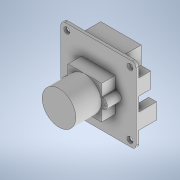
# Autodesk Inventor part: Trackingcam (Applied robotics)
Saved by Autodesk Inventor 2020 (Build 240168000, 168)
## iProperties
Created: 2021-02-21
Part Number: Trackingcam (Applied robotics)
Material: Типовые
Document SubType Name: Обычные детали
Designer: Антон
Density: 1 g/cm^3
Appearance: По умолчанию
Sheet Metal Rule: По умолчанию
Author: Антон
Autodesk Inventor part; units mm, degrees
ref_plane "YZ Plane" through (0, 0, 0) normal (1, 0, 0) x (0, 1, 0)
ref_plane "XZ Plane" through (0, 0, 0) normal (0, 1, 0) x (-1, 0, 0)
ref_plane "XY Plane" through (0, 0, 0) normal (0, 0, 1) x (1, 0, 0)
sketch "Эскиз1" plane through (0, 0, 0) normal (0, 0, 1) x (1, 0, 0)
  line L0 (0, 0) -> (38, 0)
  line L1 (38, 0) -> (38, 38)
  line L2 (38, 38) -> (0, 38)
  line L3 (0, 38) -> (0, 0)
  line L4 (0, 38) -> (3, 38)
  line L5 (3, 38) -> (3, 35)
  circle A0 centre (3, 35) radius 1.5
  circle A1 centre (35, 35) radius 1.5
  circle A2 centre (3, 3) radius 1.5
  circle A3 centre (35, 3) radius 1.5
  dimension "d0" = 38
  dimension "d1" = 38
  dimension "d2" = 3
  dimension "d3" = 3
  dimension "d4" = 3
  dimension "d7" = 32
  dimension "d10" = 32
  constraints: 12 end point, 4 centre point, 2 horizontal, 2 parallel, 2 perpendicular, 1 coincident, 1 point on line, 1 vertical, 6 other
  measures "d0" distance of L2.end L1.end
  measures "d1" distance of L1.end L0.end
  measures "d2" distance of L2.end L4.end
  measures "d3" distance of L4.end L5.end
  measures "d4" diameter of A0
  measures "d7" distance of A0.centre A1.centre
  measures "d10" distance of A0.centre A2.centre
extrude "Выдавливание1" add sketch "Эскиз1" along normal blind 1.4
fillet "Сопряжение1" radius 2 4 edges at (38, 38, 0.7) (38, 0, 0.7) (0, 0, 0.7) (0, 38, 0.7)
sketch "Эскиз2" plane through (0, 0, 1.4) normal (0, 0, 1) x (1, 0, 0)
  line L0 (2, 38) -> (10.5, 38)
  line L1 (36, 38) -> (2, 38) projected
  line L2 (10.5, 38) -> (10.5, 27.5)
  line L3 (10.5, 27.5) -> (27.5, 27.5)
  line L4 (27.5, 27.5) -> (27.5, 10.5)
  line L5 (27.5, 10.5) -> (10.5, 10.5)
  line L6 (10.5, 10.5) -> (10.5, 27.5)
  line L7 (27.5, 27.5) -> (27.5, 21.5)
  line L8 (27.5, 21.5) -> (30.5, 21.5)
  line L9 (30.5, 21.5) -> (30.5, 16.5)
  line L10 (30.5, 16.5) -> (27.5, 16.5)
  line L11 (27.5, 16.5) -> (27.5, 21.5)
  line L12 (10.5, 27.5) -> (10.5, 21.5)
  line L13 (10.5, 21.5) -> (7.5, 21.5)
  line L14 (7.5, 21.5) -> (7.5, 16.5)
  line L15 (7.5, 16.5) -> (10.5, 16.5)
  line L16 (10.5, 16.5) -> (10.5, 21.5)
  line L17 (30.5, 19) -> (29.5, 19)
  line L18 (7.5, 19) -> (8.5, 19)
  circle A0 centre (8.5, 19) radius 0.5
  circle A1 centre (29.5, 19) radius 0.5
  point P0 (0, 0)
  dimension "d20" = 8.5
  dimension "d21" = 10.5
  dimension "d22" = 17
  dimension "d23" = 17
  dimension "d83" = 6
  dimension "d84" = 3
  dimension "d85" = 5
  dimension "d86" = 6
  dimension "d87" = 3
  dimension "d88" = 5
  dimension "d89" = 1
  dimension "d90" = 1
  dimension "d91" = 1
  dimension "d92" = 1
  constraints: 36 end point, 6 parallel, 5 horizontal, 4 perpendicular, 3 point on line, 2 centre point, 2 coincident, 2 midpoint
  measures "d20" distance of L0.start L0.end
  measures "d21" distance of L0.end L2.end
  measures "d22" distance of L4.end L5.end
  measures "d23" distance of L3.end L4.end
  measures "d83" distance of L3.end L7.end
  measures "d84" distance of L9.end L10.end
  measures "d85" distance of L8.end L9.end
  measures "d86" distance of L2.end L12.end
  measures "d87" distance of L15.end L14.end
  measures "d88" distance of L14.end L13.end
  measures "d89" distance of L17.start L17.end
  measures "d90" distance of L18.start L18.end
  measures "d91" diameter of A0
  measures "d92" diameter of A1
extrude "Выдавливание2" add sketch "Эскиз2" along normal blind 7
sketch "Эскиз3" plane through (0, 0, 8.4) normal (0, 0, 1) x (1, 0, 0)
  line L0 (10.5, 27.5) -> (10.5, 10.5) projected
  line L1 (10.5, 19) -> (27.5, 19)
  line L2 (27.5, 27.5) -> (27.5, 10.5) projected
  circle A0 centre (19, 19) radius 8.5
  point P0 (0, 0)
  constraints: 3 midpoint, 2 end point, 1 horizontal alignment, 2 other
extrude "Выдавливание3" add sketch "Эскиз3" along normal blind 13
sketch "Эскиз4" plane through (0, 0, 0) normal (0, 0, -1) x (-1, 0, 0)
  arc A0 (-36, 38) -> (-38, 36) centre (-36, 36) ccw projected
  line L0 (-36, 38) -> (-29.25, 38)
  line L1 (-29.25, 38) -> (-29.25, 36)
  line L2 (-29.25, 36) -> (-8.75, 36)
  line L3 (-8.75, 36) -> (-8.75, 27)
  line L4 (-8.75, 27) -> (-29.25, 27)
  line L5 (-29.25, 27) -> (-29.25, 36)
  point P0 (0, 0)
  dimension "d41" = 6.75
  dimension "d42" = 2
  dimension "d43" = 20.5
  dimension "d44" = 9
  constraints: 12 end point, 2 horizontal, 2 parallel, 1 perpendicular, 1 tangent, 1 vertical
  measures "d41" distance of L0.start L0.end
  measures "d42" distance of L0.end L1.end
  measures "d43" distance of L3.end L4.end
  measures "d44" distance of L2.end L3.end
extrude "Выдавливание4" add sketch "Эскиз4" along normal blind 10
sketch "Эскиз5" plane through (0, 0, 0) normal (0, 0, -1) x (-1, 0, 0)
  arc A0 (-36, 38) -> (-38, 36) centre (-36, 36) ccw projected
  line L0 (-38, 36) -> (-38, 31)
  arc A1 (0, 36) -> (-2, 38) centre (-2, 36) ccw projected
  line L1 (-38, 31) -> (-33, 31)
  line L2 (-33, 31) -> (-33, 21)
  line L3 (-33, 21) -> (-38, 21)
  line L4 (-38, 21) -> (-38, 31)
  line L5 (-5, 31) -> (0, 31)
  line L6 (0, 31) -> (0, 21)
  line L7 (0, 21) -> (-5, 21)
  line L8 (-5, 21) -> (-5, 31)
  point P0 (0, 0)
  dimension "d47" = 5
  dimension "d49" = 5
  dimension "d50" = 10
  dimension "d53" = 33
  constraints: 18 end point, 2 horizontal, 2 parallel, 1 collinear, 1 perpendicular, 1 tangent, 1 vertical, 7 other
  measures "d47" distance of L0.start L0.end
  measures "d49" distance of L2.end L3.end
  measures "d50" distance of L1.end L2.end
  measures "d53" distance of L0.end L5.start
extrude "Выдавливание5" add sketch "Эскиз5" along normal blind 6
chamfer "Фаска1" distance 2 angle 45 2 edges at (38, 21, -3) (0, 31, -3)
sketch "Эскиз6" plane through (0, 0, 0) normal (0, 0, -1) x (-1, 0, 0)
  line L0 (-38, 2) -> (-38, 23) projected
  line L1 (-38, 2) -> (-38, 8)
  line L2 (-38, 8) -> (-34, 8)
  line L3 (-34, 8) -> (-34, 16)
  line L4 (-34, 16) -> (-38, 16)
  line L5 (-38, 16) -> (-38, 8)
  point P0 (0, 0)
  dimension "d63" = 6
  dimension "d64" = 4
  dimension "d65" = 8
  constraints: 10 end point, 2 parallel, 1 horizontal, 1 perpendicular, 1 point on line
  measures "d63" distance of L0.start L1.end
  measures "d64" distance of L4.end L3.end
  measures "d65" distance of L3.end L2.end
extrude "Выдавливание6" add sketch "Эскиз6" along normal blind 9
sketch "Эскиз7" plane through (0, 0, 0) normal (0, 0, -1) x (-1, 0, 0)
  line L0 (-38, 2) -> (-38, 36) projected
  line L1 (-38, 2) -> (-38, 14)
  line L2 (-38, 14) -> (-32, 14)
  line L3 (-32, 14) -> (-22, 14) construction
  line L4 (-30, 12) -> (-24, 12)
  line L5 (-24, 16) -> (-30, 16)
  arc A0 (-30, 16) -> (-30, 12) centre (-30, 14) ccw
  arc A1 (-24, 12) -> (-24, 16) centre (-24, 14) ccw
  point P0 (0, 0)
  point P1 (-27, 14)
  dimension "d68" = 12
  dimension "d69" = 6
  dimension "d70" = 10
  dimension "d71" = 4
  constraints: 12 end point, 6 point on circle, 4 tangent, 3 point on line, 2 centre point, 1 horizontal, 1 midpoint, 1 parallel, 1 perpendicular
  measures "d68" distance of L0.start L1.end
  measures "d69" distance of L1.end L2.end
  measures "d70" distance of L2.end L3.end
  measures "d71" diameter of A1
extrude "Выдавливание7" add sketch "Эскиз7" along normal blind 3
sketch "Эскиз8" plane through (0, 0, 0) normal (0, 0, -1) x (-1, 0, 0)
  arc A0 (-38, 2) -> (-36, 0) centre (-36, 2) ccw projected
  line L0 (-38, 2) -> (-38, 17)
  line L1 (-38, 17) -> (-24, 17)
  line L2 (-24, 17) -> (-18, 17)
  line L3 (-18, 17) -> (-18, 23)
  line L4 (-18, 23) -> (-24, 23)
  line L5 (-24, 23) -> (-24, 17)
  point P0 (0, 0)
  dimension "d74" = 15
  dimension "d75" = 14
  dimension "d76" = 6
  dimension "d77" = 6
  constraints: 12 end point, 2 parallel, 2 perpendicular, 1 horizontal, 1 tangent, 1 vertical
  measures "d74" distance of L0.start L0.end
  measures "d75" distance of L0.end L1.end
  measures "d76" distance of L4.end L3.end
  measures "d77" distance of L3.end L2.end
extrude "Выдавливание8" add sketch "Эскиз8" along normal blind 3.5
sketch "Эскиз9" plane through (0, 0, -3.5) normal (0, 0, -1) x (-1, 0, 0)
  line L0 (-24, 17) -> (-18, 17) projected
  line L1 (-21, 17) -> (-21, 23)
  line L2 (-24, 23) -> (-18, 23) projected
  circle A0 centre (-21, 20) radius 1.75
  point P0 (0, 0)
  dimension "d80" = 3.5
  constraints: 3 midpoint, 2 end point, 1 centre point
  measures "d80" diameter of A0
extrude "Выдавливание9" add sketch "Эскиз9" along normal blind 4
sketch "Эскиз11" plane through (0, 0, 0) normal (0, 0, -1) x (-1, 0, 0)
  circle A0 centre (-29.5, 19) radius 0.5 projected
  circle A1 centre (-8.5, 19) radius 0.5 projected
  circle A2 centre (-8.5, 19) radius 1.75
  circle A3 centre (-29.5, 19) radius 1.75
  point P0 (0, 0)
  dimension "d93" = 3.5
  dimension "d94" = 3.5
  constraints: 2 centre point, 2 coincident
  measures "d93" diameter of A2
  measures "d94" diameter of A3
extrude "Выдавливание10" add sketch "Эскиз11" along normal blind 1.5 contours A0 | A1 | A2 | A3
sketch "Эскиз12" plane through (0, 0, 1.4) normal (0, 0, 1) x (1, 0, 0)
  line L0 (0, 0) -> (0, 6.7)
  line L1 (0, 36) -> (0, 2) projected
  line L2 (0, 6.7) -> (3.7, 6.7)
  line L3 (3.7, 6.7) -> (7, 6.7)
  line L4 (7, 6.7) -> (7, 9.5)
  line L5 (7, 9.5) -> (3.7, 9.5)
  line L6 (3.7, 9.5) -> (3.7, 6.7)
  dimension "d97" = 6.7
  dimension "d98" = 3.7
  dimension "d99" = 3.3
  dimension "d100" = 2.8
  constraints: 12 end point, 2 horizontal, 2 parallel, 1 perpendicular, 1 point on line
  measures "d97" distance of L0.start L0.end
  measures "d98" distance of L0.end L2.end
  measures "d99" distance of L5.end L4.end
  measures "d100" distance of L4.end L3.end
extrude "Выдавливание11" add sketch "Эскиз12" along normal blind 2
fillet "Сопряжение2" radius 2.5 4 edges at (7.5, 16.5, 4.9) (7.5, 21.5, 4.9) (30.5, 21.5, 4.9) (30.5, 16.5, 4.9)
equation "\"d3\" = d2"
equation "\"Радиус_гибки\" = Толщина"
equation "\"Ширина_просечки\" = Толщина"
equation "\"Глубина_просечки\" = 0.5 * Толщина"
equation "\"Размер_просечки\" = 4 * Толщина"
equation "\"Мин_остаток\" = 2 * Толщина"
equation "\"Радиус_перехода\" = Радиус_гибки"
equation "\"Радиус_Якоби\" = Толщина"
equation "\"Размер_зазора\" = Толщина"
equation "\"Толщина\" = 0.5"
